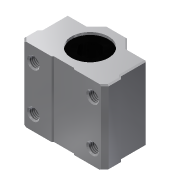
# Autodesk Inventor part: SV8UU
Saved by Autodesk Inventor 2014 (Build 180170000, 170)
## iProperties
Created: 2014-07-29
Part Number: SV8UU
Material: Generic
Document SubType Name: Modeling
Designer: ntg
Density: 1 g/cm^3
Appearance: Aluminum - Polished
Author: ntg
Autodesk Inventor part; units mm, degrees
ref_plane "YZ Plane" through (0, 0, 0) normal (1, 0, 0) x (0, 1, 0)
ref_plane "XZ Plane" through (0, 0, 0) normal (0, 1, 0) x (-1, 0, 0)
ref_plane "XY Plane" through (0, 0, 0) normal (0, 0, 1) x (1, 0, 0)
sketch "Sketch1" plane through (0, 0, 0) normal (0, 0, 1) x (1, 0, 0)
  line L0 (-15.9064, 9.3186) -> (-7.9064, 9.3186)
  line L1 (-7.9064, 9.3186) -> (-3.9064, 13.3186)
  line L2 (-3.9064, 13.3186) -> (4.0936, 13.3186)
  line L3 (4.0936, 13.3186) -> (8.0936, 9.3186)
  line L4 (8.0936, 9.3186) -> (16.0936, 9.3186)
  line L5 (-15.9064, 9.3186) -> (-15.9064, -1.1814)
  line L6 (-15.9064, -1.1814) -> (-16.9064, -2.1814)
  line L7 (-16.9064, -2.1814) -> (-16.9064, -7.1814)
  line L8 (-16.9064, -7.1814) -> (-15.9064, -8.1814)
  line L9 (16.0936, 9.3186) -> (16.0936, -1.1814)
  line L10 (16.0936, -1.1814) -> (17.0936, -2.1814)
  line L11 (17.0936, -2.1814) -> (17.0936, -7.1814)
  line L12 (17.0936, -7.1814) -> (16.0936, -8.1814)
  line L13 (16.0936, -8.1814) -> (-15.9064, -8.1814) construction
  line L14 (-15.9064, -8.6814) -> (16.0936, -8.6814) construction
  line L15 (-15.9064, -8.1814) -> (-15.4064, -8.6814)
  line L16 (-15.4064, -8.6814) -> (-4.4064, -8.6814)
  line L17 (-4.4064, -8.6814) -> (-3.9064, -8.1814)
  line L18 (-3.9064, -8.1814) -> (4.0936, -8.1814)
  line L19 (4.0936, -8.1814) -> (4.5936, -8.6814)
  line L20 (16.0936, -8.1814) -> (15.5936, -8.6814)
  line L21 (15.5936, -8.6814) -> (4.5936, -8.6814)
  line L22 (-11.9064, 9.3186) -> (-11.9064, 8.0705)
  dimension "d23" = 8
  dimension "d24" = 135
  dimension "d25" = 135
  dimension "d26" = 4
  dimension "d27" = 8
  dimension "d28" = 8
  dimension "d29" = 135
  dimension "d30" = 135
  dimension "d31" = 10.5
  dimension "d32" = 135
  dimension "d33" = 135
  dimension "d34" = 1
  dimension "d35" = 1
  dimension "d36" = 135
  dimension "d37" = 135
  dimension "d38" = 135
  dimension "d39" = 1
  dimension "d40" = 10.5
  dimension "d41" = 5
  dimension "d42" = 5
  dimension "d136" = 0.5
  dimension "d137" = 11
  dimension "d138" = 8
  dimension "d139" = 135
  dimension "d140" = 135
  dimension "d141" = 135
  dimension "d142" = 135
  dimension "d143" = 135
  dimension "d144" = 11
  constraints: 46 end point, 7 point on line, 1 midpoint
  measures "d23" distance of L0.start L0.end
  measures "d24" angle of L0 L1
  measures "d25" angle of L2 L1
  measures "d26" distance from line of L0.end L2
  measures "d27" distance of L1.end L2.end
  measures "d28" distance of L3.end L4.end
  measures "d29" angle of L2 L3
  measures "d30" angle of L3 L4
  measures "d31" distance of L0.start L5.end
  measures "d32" angle of L5 L6
  measures "d33" angle of L7 L6
  measures "d34" distance from line of L5.end L7
  measures "d35" distance from line of L9.end L11
  measures "d36" angle of L9 L10
  measures "d37" angle of L10 L11
  measures "d38" angle of L11 L12
  measures "d39" distance from line of L11 L12.end
  measures "d40" distance of L4.end L9.end
  measures "d41" distance of L6.end L7.end
  measures "d42" distance of L10.end L11.end
  measures "d136" distance between parallel lines of L13 L14
  measures "d137" distance of L15.end L16.end
  measures "d138" distance of L17.end L18.end
  measures "d139" angle of L13 L19
  measures "d140" angle of L14 L19
  measures "d141" angle of L14 L20
  measures "d142" angle of L16 L17
  measures "d143" angle of L15 L16
  measures "d144" distance of L20.end L19.end
extrude "Extrusion1" add sketch "Sketch1" along normal blind 30
hole "Hole1" at (0.0936, 2.3186, 30) direction (0, 0, -1) diameter 15 depth 1
hole "Hole2" at (0.0936, 2.3186, 0) direction (0, 0, 1) diameter 15 depth 1
hole "Hole3" at (0.0936, 2.3186, 1) direction (0, 0, 1) diameter 8.05 depth 28
chamfer "Chamfer5" distance 0.5 angle 45 28 edges at (-16.1564, -7.9314, 30) (-16.9064, -4.6814, 30) (-16.4064, -1.6814, 30) (-15.9064, 4.0686, 30) (-11.9064, 9.3186, 30) (-5.9064, 11.3186, 30) (0.0936, 13.3186, 30) (6.0936, 11.3186, 30) (12.0936, 9.3186, 30) (16.0936, 4.0686, 30) (16.5936, -1.6814, 30) (17.0936, -4.6814, 30) (16.3436, -7.9314, 30) (16.0936, 9.3186, 15) (16.3436, -7.9314, 0) (17.0936, -4.6814, 0) (16.5936, -1.6814, 0) (16.0936, 4.0686, 0) (12.0936, 9.3186, 0) (6.0936, 11.3186, 0) (0.0936, 13.3186, 0) (-5.9064, 11.3186, 0) (-11.9064, 9.3186, 0) (-15.9064, 4.0686, 0) (-16.4064, -1.6814, 0) (-16.9064, -4.6814, 0) (-16.1564, -7.9314, 0) (-15.9064, 9.3186, 15)
hole "Hole8" at (12.0936, -8.6814, 6) direction (0, 1, 0) diameter 4 depth 18 countersink diameter 5 countersink angle 90
hole "Hole9" at (12.0936, -8.6814, 24) direction (0, 1, 0) diameter 4 depth 18 countersink diameter 5 countersink angle 90
hole "Hole10" at (-11.9064, -8.6814, 24) direction (0, 1, 0) diameter 4 depth 18 countersink diameter 5 countersink angle 90
hole "Hole11" at (-11.9064, -8.6814, 6) direction (0, 1, 0) diameter 4 depth 18 countersink diameter 5 countersink angle 90
hole "Hole12" at (-11.9064, 9.3186, 24) direction (0, -1, 0) diameter 4 depth 18 countersink diameter 5 countersink angle 90
hole "Hole13" at (-11.9064, 9.3186, 6) direction (0, -1, 0) diameter 4 depth 18 countersink diameter 5 countersink angle 90
hole "Hole14" at (12.0936, 9.3186, 6) direction (0, -1, 0) diameter 4 depth 18 countersink diameter 5 countersink angle 90
hole "Hole15" at (12.0936, 9.3186, 24) direction (0, -1, 0) diameter 4 depth 18 countersink diameter 5 countersink angle 90
thread "Thread1" size "M4x0.7" class "6H" standard "ANSI Metric M Profile" full length
thread "Thread2" size "M4x0.7" class "6H" standard "ANSI Metric M Profile" full length
thread "Thread3" size "M4x0.7" class "6H" standard "ANSI Metric M Profile" full length
thread "Thread4" size "M4x0.7" class "6H" standard "ANSI Metric M Profile" full length
equation "\"d37\" = d36"
equation "\"d38\" = d36"
equation "\"d40\" = d31"
body "Solid1"
